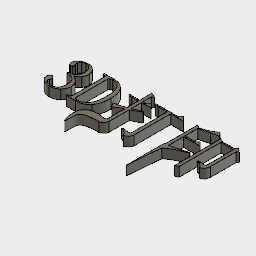
艺术字 (Autodesk Fusion 360 design; units mm, degrees)
Autodesk Fusion 360 part; units mm, degrees
sketch "草图1" plane through (0, 0, 0) normal (0, 1, 0) x (1, 0, 0)
  line L0 (23.9944, 3.8481) -> (23.9944, 4.5512)
  line L1 (37.5881, 11.9341) -> (37.5881, -4.8238)
  line L2 (34.728, 12.8716) -> (34.0725, 12.8716)
  line L3 (34.0725, 12.8716) -> (34.0725, 13.5747)
  line L4 (34.0725, 13.5747) -> (39.3002, 13.5747)
  line L5 (39.0237, -6.4644) -> (34.0725, -6.4644)
  line L6 (34.0725, -6.4644) -> (34.0725, -5.7613)
  line L7 (34.0725, -5.7613) -> (34.7903, -5.7613)
  line L8 (35.7131, -4.8238) -> (35.7131, 11.9341)
  line L9 (68.2912, -5.9956) -> (68.2912, 12.6372)
  line L10 (68.2912, 12.6372) -> (63.4866, 12.6372)
  line L11 (63.4866, 12.6372) -> (62.1975, 12.4028)
  line L12 (62.1975, 12.4028) -> (61.26, 13.3403)
  line L13 (61.26, 13.3403) -> (73.0959, 13.3403)
  line L14 (73.0959, 13.3403) -> (74.6194, 14.8637)
  line L15 (74.6194, 14.8637) -> (76.8459, 12.6372)
  line L16 (76.8459, 12.6372) -> (70.0491, 12.6372)
  line L17 (70.0491, 12.6372) -> (70.0491, -6.6988)
  line L18 (63.8381, -7.0503) -> (63.8381, -6.4644)
  line L19 (55.635, 4.0825) -> (55.635, 10.0591)
  line L20 (55.635, 10.0591) -> (52.1194, 10.0591)
  line L21 (52.1194, 10.0591) -> (50.8303, 9.8247)
  line L22 (50.8303, 9.8247) -> (49.8928, 10.7622)
  line L23 (49.8928, 10.7622) -> (55.635, 10.7622)
  line L24 (55.5178, 17.2075) -> (58.2131, 16.0356)
  line L25 (58.2131, 16.0356) -> (57.2756, 15.2153)
  line L26 (57.2756, 15.2153) -> (57.2756, 10.7622)
  line L27 (57.2756, 10.7622) -> (59.0334, 10.7622)
  line L28 (59.0334, 10.7622) -> (60.3225, 12.0512)
  line L29 (60.3225, 12.0512) -> (62.3147, 10.0591)
  line L30 (62.3147, 10.0591) -> (57.2756, 10.0591)
  line L31 (57.2756, 10.0591) -> (57.2756, 4.6684)
  line L32 (57.2756, 4.6684) -> (61.8459, 6.5434)
  line L33 (61.8459, 6.5434) -> (62.0803, 6.0747)
  line L34 (62.0803, 6.0747) -> (57.2756, 3.4966)
  line L35 (57.2756, 3.4966) -> (57.2756, -7.0503)
  line L36 (55.635, -5.6441) -> (55.635, 2.7934)
  line L37 (51.4162, 0.2153) -> (49.8928, 2.3247)
  line L38 (102.9787, -0.605) -> (102.9787, 12.8716)
  line L39 (102.9787, 12.8716) -> (96.2991, 12.8716)
  line L40 (96.2991, 12.8716) -> (96.2991, -9.1597)
  line L41 (96.2991, -9.1597) -> (94.5412, -9.98)
  line L42 (94.6584, -6.5816) -> (94.6584, 11.1137)
  line L43 (94.5412, 14.6294) -> (96.1819, 13.5747)
  line L44 (96.1819, 13.5747) -> (102.7444, 13.5747)
  line L45 (102.7444, 13.5747) -> (103.5647, 14.8637)
  line L46 (103.5647, 14.8637) -> (105.5569, 13.3403)
  line L47 (105.5569, 13.3403) -> (104.6194, 12.52)
  line L48 (104.6194, 12.52) -> (104.6194, -0.9566)
  line L49 (98.6428, -2.0113) -> (98.76, -1.5425)
  line L50 (82.2366, -1.1909) -> (82.2366, 11.8169)
  line L51 (82.1194, 14.7466) -> (83.8772, 13.6919)
  line L52 (91.4944, 17.3247) -> (93.2522, 15.2153)
  line L53 (83.8772, 13.1059) -> (83.8772, 6.3091)
  line L54 (83.8772, 6.3091) -> (89.1506, 6.3091)
  line L55 (89.1506, 6.3091) -> (90.5569, 7.7153)
  line L56 (90.5569, 7.7153) -> (92.6662, 5.6059)
  line L57 (92.6662, 5.6059) -> (83.8772, 5.6059)
  line L58 (83.8772, 5.6059) -> (83.8772, -2.48)
  line L59 (83.8772, -2.48) -> (92.9006, 0.0981)
  line L60 (92.9006, 0.0981) -> (93.0178, -0.3706)
  spline S0 degree 3 poles (31.3772, -1.1159) (31.3042, -1.8355) (31.1555, -3.3003) (30.215, -4.4351) (29.7366, -5.0123) knots 0 0 0 0 0.211923 0.431393 0.431393 0.431393 0.431393
  spline S1 degree 3 poles (29.7366, -5.0123) (29.109, -5.5037) (27.7717, -6.5509) (26.0696, -6.6475) (25.1662, -6.6988) knots 0 0 0 0 0.233509 0.497638 0.497638 0.497638 0.497638
  spline S2 degree 3 poles (25.1662, -6.6988) (24.4943, -6.655) (23.1834, -6.5697) (22.0741, -5.8686) (21.5334, -5.5269) knots 0 0 0 0 0.198463 0.387173 0.387173 0.387173 0.387173
  spline S3 degree 3 poles (21.5334, -5.5269) (21.0897, -5.1411) (20.2585, -4.4185) (20.089, -3.3361) (20.01, -2.8316) knots 0 0 0 0 0.170073 0.318594 0.318594 0.318594 0.318594
  spline S4 degree 3 poles (20.01, -2.8316) (20.0284, -2.6049) (20.065, -2.1535) (20.3278, -1.7847) (20.4586, -1.6011) knots 0 0 0 0 0.066865 0.133166 0.133166 0.133166 0.133166
  spline S5 degree 3 poles (20.4586, -1.6011) (20.5964, -1.448) (20.842, -1.1753) (21.1991, -1.1047) (21.3558, -1.0738) knots 0 0 0 0 0.059806 0.106564 0.106564 0.106564 0.106564
  spline S6 degree 3 poles (21.3558, -1.0738) (21.5619, -1.0933) (21.9617, -1.1313) (22.195, -1.4564) (22.308, -1.6139) knots 0 0 0 0 0.058971 0.114386 0.114386 0.114386 0.114386
  spline S7 degree 3 poles (22.308, -1.6139) (22.3892, -1.7757) (22.5326, -2.0613) (22.5713, -2.3777) (22.5881, -2.5148) knots 0 0 0 0 0.053802 0.094961 0.094961 0.094961 0.094961
  spline S8 degree 3 poles (22.5881, -2.5148) (22.5809, -2.7028) (22.5671, -3.0581) (22.422, -3.3821) (22.3537, -3.5347) knots 0 0 0 0 0.055835 0.105512 0.105512 0.105512 0.105512
  spline S9 degree 3 poles (22.3537, -3.5347) (22.2855, -3.6668) (22.1585, -3.9126) (22.1318, -4.1875) (22.1194, -4.3147) knots 0 0 0 0 0.044119 0.08211 0.08211 0.08211 0.08211
  spline S10 degree 3 poles (22.1194, -4.3147) (22.1697, -4.5517) (22.2821, -5.0805) (22.7513, -5.361) (23.0102, -5.5159) knots 0 0 0 0 0.069752 0.155667 0.155667 0.155667 0.155667
  spline S11 degree 3 poles (23.0102, -5.5159) (23.3174, -5.6558) (23.9414, -5.94) (24.6263, -5.9769) (24.974, -5.9956) knots 0 0 0 0 0.100311 0.203753 0.203753 0.203753 0.203753
  spline S12 degree 3 poles (24.974, -5.9956) (25.6283, -5.9614) (26.8445, -5.8979) (27.7675, -5.1131) (28.1939, -4.7505) knots 0 0 0 0 0.19036 0.353848 0.353848 0.353848 0.353848
  spline S13 degree 3 poles (28.1939, -4.7505) (28.5059, -4.235) (29.2185, -3.0575) (29.2501, -1.6739) (29.2678, -0.8961) knots 0 0 0 0 0.177893 0.406299 0.406299 0.406299 0.406299
  spline S14 degree 3 poles (29.2678, -0.8961) (29.2336, -0.234) (29.169, 1.0155) (28.4789, 2.0549) (28.1545, 2.5435) knots 0 0 0 0 0.194741 0.367482 0.367482 0.367482 0.367482
  spline S15 degree 3 poles (28.1545, 2.5435) (27.6406, 2.9216) (26.4174, 3.8215) (24.8837, 3.8384) (23.9944, 3.8481) knots 0 0 0 0 0.187264 0.445678 0.445678 0.445678 0.445678
  spline S16 degree 3 poles (23.9944, 4.5512) (24.6814, 4.5758) (25.9268, 4.6204) (26.9181, 5.3628) (27.3626, 5.6957) knots 0 0 0 0 0.200424 0.363322 0.363322 0.363322 0.363322
  spline S17 degree 3 poles (27.3626, 5.6957) (27.6786, 6.1366) (28.3599, 7.0873) (28.4169, 8.2601) (28.4475, 8.889) knots 0 0 0 0 0.159388 0.343676 0.343676 0.343676 0.343676
  spline S18 degree 3 poles (28.4475, 8.889) (28.4155, 9.4278) (28.353, 10.4783) (27.8372, 11.3944) (27.586, 11.8407) knots 0 0 0 0 0.159572 0.311093 0.311093 0.311093 0.311093
  spline S19 degree 3 poles (27.586, 11.8407) (27.2431, 12.2094) (26.5179, 12.9892) (25.4505, 13.0656) (24.8879, 13.1059) knots 0 0 0 0 0.145675 0.308064 0.308064 0.308064 0.308064
  spline S20 degree 3 poles (24.8879, 13.1059) (24.6068, 13.0846) (24.0085, 13.0391) (23.4542, 12.8081) (23.1603, 12.6857) knots 0 0 0 0 0.084041 0.178813 0.178813 0.178813 0.178813
  spline S21 degree 3 poles (23.1603, 12.6857) (22.8909, 12.5261) (22.3616, 12.2126) (22.2777, 11.6046) (22.2366, 11.306) knots 0 0 0 0 0.088774 0.174412 0.174412 0.174412 0.174412
  spline S22 degree 3 poles (22.2366, 11.306) (22.2304, 11.0395) (22.2207, 10.6181) (22.4037, 10.2428) (22.4709, 10.1048) knots 0 0 0 0 0.078314 0.123865 0.123865 0.123865 0.123865
  spline S23 degree 3 poles (22.4709, 10.1048) (22.5393, 10.0187) (22.6788, 9.8427) (22.6964, 9.6186) (22.7053, 9.5043) knots 0 0 0 0 0.032225 0.065791 0.065791 0.065791 0.065791
  spline S24 degree 3 poles (22.7053, 9.5043) (22.6995, 9.3206) (22.6888, 8.9831) (22.5392, 8.6814) (22.4709, 8.5439) knots 0 0 0 0 0.054356 0.099886 0.099886 0.099886 0.099886
  spline S25 degree 3 poles (22.4709, 8.5439) (22.3704, 8.4392) (22.1489, 8.2084) (21.8267, 8.1927) (21.6506, 8.1841) knots 0 0 0 0 0.042033 0.092643 0.092643 0.092643 0.092643
  spline S26 degree 3 poles (21.6506, 8.1841) (21.4944, 8.2009) (21.1692, 8.2358) (20.9076, 8.4331) (20.7717, 8.5356) knots 0 0 0 0 0.046253 0.096251 0.096251 0.096251 0.096251
  spline S27 degree 3 poles (20.7717, 8.5356) (20.6528, 8.6958) (20.3718, 9.0743) (20.3653, 9.5502) (20.3616, 9.8247) knots 0 0 0 0 0.058539 0.138302 0.138302 0.138302 0.138302
  spline S28 degree 3 poles (20.3616, 9.8247) (20.4302, 10.3875) (20.5704, 11.5371) (21.4407, 12.3042) (21.885, 12.6958) knots 0 0 0 0 0.164147 0.335309 0.335309 0.335309 0.335309
  spline S29 degree 3 poles (21.885, 12.6958) (22.4171, 13.0205) (23.497, 13.6795) (24.7599, 13.7655) (25.4006, 13.8091) knots 0 0 0 0 0.184087 0.373642 0.373642 0.373642 0.373642
  spline S30 degree 3 poles (25.4006, 13.8091) (26.1327, 13.7577) (27.5417, 13.659) (28.6285, 12.7622) (29.1506, 12.3314) knots 0 0 0 0 0.214148 0.412134 0.412134 0.412134 0.412134
  spline S31 degree 3 poles (29.1506, 12.3314) (29.5604, 11.8494) (30.3349, 10.9381) (30.4858, 9.7555) (30.5569, 9.1985) knots 0 0 0 0 0.185177 0.350055 0.350055 0.350055 0.350055
  spline S32 degree 3 poles (30.5569, 9.1985) (30.5267, 8.6386) (30.4687, 7.5632) (29.9342, 6.63) (29.678, 6.1827) knots 0 0 0 0 0.165573 0.318027 0.318027 0.318027 0.318027
  spline S33 degree 3 poles (29.678, 6.1827) (29.3243, 5.7903) (28.5647, 4.9473) (27.4955, 4.5579) (26.9241, 4.3498) knots 0 0 0 0 0.156088 0.335315 0.335315 0.335315 0.335315
  spline S34 degree 3 poles (26.9241, 4.3498) (27.6903, 4.0515) (29.0642, 3.5164) (30.0179, 2.4007) (30.4397, 1.9072) knots 0 0 0 0 0.242019 0.433971 0.433971 0.433971 0.433971
  spline S35 degree 3 poles (30.4397, 1.9072) (30.713, 1.415) (31.2369, 0.4715) (31.3318, -0.6022) (31.3772, -1.1159) knots 0 0 0 0 0.166749 0.319663 0.319663 0.319663 0.319663
  spline S36 degree 3 poles (45.0881, 3.7309) (45.0829, 5.1921) (45.074, 7.6802) (43.9888, 9.9032) (43.5409, 10.8208) knots 0 0 0 0 0.430939 0.733834 0.733834 0.733834 0.733834
  spline S37 degree 3 poles (43.5409, 10.8208) (42.9671, 11.4189) (41.7976, 12.638) (40.1127, 12.7927) (39.2544, 12.8716) knots 0 0 0 0 0.240222 0.489672 0.489672 0.489672 0.489672
  spline S38 degree 3 poles (39.2544, 12.8716) (39.008, 12.8687) (38.5763, 12.8637) (38.1763, 12.7052) (38.0047, 12.6372) knots 0 0 0 0 0.073134 0.128092 0.128092 0.128092 0.128092
  spline S39 degree 3 poles (38.0047, 12.6372) (37.8832, 12.5498) (37.6417, 12.376) (37.6059, 12.0808) (37.5881, 11.9341) knots 0 0 0 0 0.04283 0.085147 0.085147 0.085147 0.085147
  spline S40 degree 3 poles (37.5881, -4.8238) (37.6013, -4.9691) (37.6268, -5.2518) (37.8411, -5.4369) (37.9452, -5.5269) knots 0 0 0 0 0.041976 0.081667 0.081667 0.081667 0.081667
  spline S41 degree 3 poles (37.9452, -5.5269) (38.0815, -5.5951) (38.3804, -5.7446) (38.7152, -5.7554) (38.8973, -5.7613) knots 0 0 0 0 0.045213 0.099091 0.099091 0.099091 0.099091
  spline S42 degree 3 poles (38.8973, -5.7613) (39.7363, -5.6803) (41.4164, -5.5181) (42.6735, -4.3916) (43.3028, -3.8277) knots 0 0 0 0 0.245947 0.492507 0.492507 0.492507 0.492507
  spline S43 degree 3 poles (43.3028, -3.8277) (43.8186, -2.8945) (45.1067, -0.5641) (45.0951, 2.121) (45.0881, 3.7309) knots 0 0 0 0 0.315469 0.787798 0.787798 0.787798 0.787798
  spline S44 degree 3 poles (35.7131, 11.9341) (35.7085, 12.0753) (35.7, 12.3312) (35.558, 12.5425) (35.4943, 12.6372) knots 0 0 0 0 0.041379 0.074959 0.074959 0.074959 0.074959
  spline S45 degree 3 poles (35.4943, 12.6372) (35.3972, 12.7052) (35.1693, 12.8647) (34.8889, 12.869) (34.728, 12.8716) knots 0 0 0 0 0.034855 0.081754 0.081754 0.081754 0.081754
  spline S46 degree 3 poles (39.3002, 13.5747) (40.4259, 13.4916) (42.6008, 13.331) (44.2522, 11.9143) (45.0488, 11.2309) knots 0 0 0 0 0.328968 0.635524 0.635524 0.635524 0.635524
  spline S47 degree 3 poles (45.0488, 11.2309) (45.6732, 10.2628) (47.0906, 8.0653) (47.1591, 5.4361) (47.1975, 3.9653) knots 0 0 0 0 0.339513 0.770608 0.770608 0.770608 0.770608
  spline S48 degree 3 poles (47.1975, 3.9653) (47.1681, 2.3666) (47.1163, -0.4532) (45.7266, -2.8897) (45.1247, -3.9448) knots 0 0 0 0 0.47015 0.829271 0.829271 0.829271 0.829271
  spline S49 degree 3 poles (45.1247, -3.9448) (44.3157, -4.679) (42.5928, -6.2422) (40.2606, -6.3874) (39.0237, -6.4644) knots 0 0 0 0 0.318321 0.677825 0.677825 0.677825 0.677825
  spline S50 degree 3 poles (34.7903, -5.7613) (34.9415, -5.7582) (35.207, -5.753) (35.4174, -5.5949) (35.508, -5.5269) knots 0 0 0 0 0.043971 0.0772 0.0772 0.0772 0.0772
  spline S51 degree 3 poles (35.508, -5.5269) (35.5677, -5.4318) (35.7018, -5.2181) (35.7091, -4.9646) (35.7131, -4.8238) knots 0 0 0 0 0.033089 0.074424 0.074424 0.074424 0.074424
  spline S52 degree 3 poles (63.8381, -6.4644) (64.7053, -6.5974) (65.9888, -6.7944) (67.2849, -6.8549) (67.7053, -6.8745) knots 0 0 0 0 0.26291 0.389099 0.389099 0.389099 0.389099
  spline S53 degree 3 poles (67.7053, -6.8745) (67.8756, -6.8093) (68.2638, -6.6605) (68.2814, -6.2347) (68.2912, -5.9956) knots 0 0 0 0 0.050511 0.11518 0.11518 0.11518 0.11518
  spline S54 degree 3 poles (70.0491, -6.6988) (69.8914, -7.3393) (69.533, -8.7958) (68.1362, -9.4046) (67.3537, -9.7456) knots 0 0 0 0 0.188254 0.428005 0.428005 0.428005 0.428005
  spline S55 degree 3 poles (67.3537, -9.7456) (67.0673, -9.1753) (66.3514, -7.7498) (64.7805, -7.3126) (63.8381, -7.0503) knots 0 0 0 0 0.184477 0.461127 0.461127 0.461127 0.461127
  spline S56 degree 3 poles (49.8928, 2.3247) (50.5695, 2.4809) (52.523, 2.9319) (54.4049, 3.6277) (55.635, 4.0825) knots 0 0 0 0 0.208193 0.601012 0.601012 0.601012 0.601012
  spline S57 degree 3 poles (55.635, 10.7622) (55.6311, 11.8853) (55.6235, 14.0344) (55.552, 16.1822) (55.5178, 17.2075) knots 0 0 0 0 0.336927 0.64467 0.64467 0.64467 0.64467
  spline S58 degree 3 poles (57.2756, -7.0503) (57.1122, -7.6477) (56.7518, -8.9648) (55.4992, -9.5455) (54.8147, -9.8628) knots 0 0 0 0 0.177361 0.391068 0.391068 0.391068 0.391068
  spline S59 degree 3 poles (51.1819, -6.3472) (51.95, -6.5146) (53.1497, -6.7762) (54.3742, -6.8485) (54.8147, -6.8745) knots 0 0 0 0 0.235312 0.367546 0.367546 0.367546 0.367546
  spline S60 degree 3 poles (54.8147, -6.8745) (55.0529, -6.7873) (55.6024, -6.586) (55.6232, -5.9847) (55.635, -5.6441) knots 0 0 0 0 0.070144 0.161823 0.161823 0.161823 0.161823
  spline S61 degree 3 poles (55.635, 2.7934) (54.644, 2.338) (53.1311, 1.6428) (51.856, 0.5814) (51.4162, 0.2153) knots 0 0 0 0 0.325024 0.496154 0.496154 0.496154 0.496154
  spline S62 degree 3 poles (98.76, -1.5425) (99.399, -1.61) (100.4709, -1.7231) (101.5478, -1.7614) (101.9827, -1.7769) knots 0 0 0 0 0.192698 0.323201 0.323201 0.323201 0.323201
  spline S63 degree 3 poles (101.9827, -1.7769) (102.2729, -1.7166) (102.8934, -1.5876) (102.9491, -0.9464) (102.9787, -0.605) knots 0 0 0 0 0.080246 0.171597 0.171597 0.171597 0.171597
  spline S64 degree 3 poles (94.5412, -9.98) (94.5742, -9.2477) (94.6253, -8.1153) (94.6498, -6.982) (94.6584, -6.5816) knots 0 0 0 0 0.219902 0.340055 0.340055 0.340055 0.340055
  spline S65 degree 3 poles (94.6584, 11.1137) (94.6514, 11.6216) (94.6352, 12.7942) (94.5752, 13.9655) (94.5412, 14.6294) knots 0 0 0 0 0.152372 0.351784 0.351784 0.351784 0.351784
  spline S66 degree 3 poles (104.6194, -0.9566) (104.5236, -1.6927) (104.3205, -3.2539) (102.906, -3.9743) (102.1584, -4.355) knots 0 0 0 0 0.209672 0.444669 0.444669 0.444669 0.444669
  spline S67 degree 3 poles (102.1584, -4.355) (101.8991, -3.8834) (101.1679, -2.5533) (99.6333, -2.2239) (98.6428, -2.0113) knots 0 0 0 0 0.156018 0.440001 0.440001 0.440001 0.440001
  spline S68 degree 3 poles (81.7678, -3.0659) (81.9324, -2.7999) (82.2864, -2.2274) (82.2539, -1.5523) (82.2366, -1.1909) knots 0 0 0 0 0.091714 0.197345 0.197345 0.197345 0.197345
  spline S69 degree 3 poles (82.2366, 11.8169) (82.2285, 12.1978) (82.208, 13.1751) (82.1529, 14.151) (82.1194, 14.7466) knots 0 0 0 0 0.114295 0.293222 0.293222 0.293222 0.293222
  spline S70 degree 3 poles (83.8772, 13.6919) (85.5859, 14.1934) (88.3324, 14.9996) (90.6272, 16.687) (91.4944, 17.3247) knots 0 0 0 0 0.528401 0.849359 0.849359 0.849359 0.849359
  spline S71 degree 3 poles (93.2522, 15.2153) (92.6443, 15.1453) (91.2977, 14.9903) (89.9869, 14.6437) (89.2678, 14.4536) knots 0 0 0 0 0.18334 0.406116 0.406116 0.406116 0.406116
  spline S72 degree 3 poles (89.2678, 14.4536) (88.429, 14.2298) (86.6392, 13.7523) (84.8355, 13.3302) (83.8772, 13.1059) knots 0 0 0 0 0.260433 0.555682 0.555682 0.555682 0.555682
  spline S73 degree 3 poles (93.0178, -0.3706) (90.7427, -1.1463) (87.2538, -2.3357) (84.314, -4.5293) (83.2912, -5.2925) knots 0 0 0 0 0.714393 1.095534 1.095534 1.095534 1.095534
  line L61 (81.7678, -3.0659) -> (81.7678, -22.541)
  line L62 (81.7678, -22.541) -> (83.2912, -5.2925)
  spline S74 degree 5 poles (51.1819, -6.3472) (51.0819, -6.3562) (50.8823, -6.3751) (50.5837, -6.4065) (50.1869, -6.4542) (49.6937, -6.524) (49.2038, -6.6051) (48.718, -6.6994) (48.2383, -6.8102) (47.7671, -6.9427) (47.3076, -7.1024) (46.8636, -7.2947) (46.4389, -7.5233) (46.0374, -7.7895) (45.6628, -8.0914) (45.3185, -8.4249) (45.0075, -8.7849) (44.7324, -9.1665) (44.4952, -9.5662) (44.2974, -9.9823) (44.1392, -10.414) (44.0197, -10.8606) (43.9366, -11.3207) (43.8853, -11.7912) (43.8603, -12.2676) (43.8552, -12.7438) (43.8643, -13.213) (43.8829, -13.6678) (43.9084, -14.1004) (43.9404, -14.5055) (43.9809, -14.8846) (44.0341, -15.248) (44.1072, -15.6202) (44.2081, -16.0324) (44.3426, -16.5074) (44.5116, -17.048) (44.7081, -17.623) (44.9149, -18.1571) (45.1106, -18.5565) (45.2745, -18.7327) (45.3919, -18.6251) (45.4602, -18.2283) (45.4873, -17.5858) (45.4879, -16.7713) (45.4797, -15.8751) (45.4807, -14.9871) (45.5055, -14.1833) (45.5611, -13.5076) (45.6467, -12.9656) (45.7579, -12.539) (45.8909, -12.1957) (46.0459, -11.9008) (46.2321, -11.6285) (46.4686, -11.3689) (46.7766, -11.121) (47.1737, -10.8896) (47.6665, -10.6792) (48.2486, -10.4922) (48.9046, -10.3297) (49.613, -10.1916) (50.3497, -10.077) (51.0905, -9.9849) (51.8147, -9.9141) (52.5078, -9.8637) (53.1599, -9.8332) (53.7655, -9.8222) (54.2103, -9.8288) (54.5213, -9.8424) (54.7186, -9.8554) (54.8147, -9.8628) knots 0 0 0 0 0 0 0.01538462 0.03076923 0.04615385 0.06153846 0.07692308 0.09230769 0.10769231 0.12307692 0.13846154 0.15384615 0.16923077 0.18461538 0.2 0.21538462 0.23076923 0.24615385 0.26153846 0.27692308 0.29230769 0.30769231 0.32307692 0.33846154 0.35384615 0.36923077 0.38461538 0.4 0.41538462 0.43076923 0.44615385 0.46153846 0.47692308 0.49230769 0.50769231 0.52307692 0.53846154 0.55384615 0.56923077 0.58461538 0.6 0.61538462 0.63076923 0.64615385 0.66153846 0.67692308 0.69230769 0.70769231 0.72307692 0.73846154 0.75384615 0.76923077 0.78461538 0.8 0.81538462 0.83076923 0.84615385 0.86153846 0.87692308 0.89230769 0.90769231 0.92307692 0.93846154 0.95384615 0.96923077 0.98461538 1 1 1 1 1 1
  point P0 (48.724, -6.7026)
  point P1 (46.5, -7.5)
  point P2 (44.8346, -9.0344)
  point P3 (44, -11)
  point P4 (43.8675, -13.2338)
  point P5 (44, -15)
  point P6 (44.5, -17)
  point P7 (45.2958, -18.6617)
  point P8 (45.5, -14.5)
  point P9 (46, -12)
  point P10 (47, -11)
  point P11 (51, -10)
sketch "草图2" plane through (0, 0, 0) normal (0, 1, 0) x (1, 0, 0)
extrude "拉伸1" add sketch "草图1" along normal blind 5 makes body 1 at (70.0491, 1.6667, -6.1919) makes body 2 at (30.5973, 0, 1.7562) makes body 3 at (81.7678, 3.3333, 9.5576) makes body 4 at (45.4859, 0.9662, 17.0026) makes body 5 at (36.9631, 0, -0.7622) makes body 6 at (96.2991, 3.3333, -5.5278)
